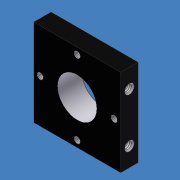
# Autodesk Inventor part: BB2-FrontPlate
Saved by Autodesk Inventor 2012 (Build 160160000, 160)
## iProperties
Company: FirstCadLibrary
Shininess: 64.0
Length Units: 11269
Angle Units: 11279
Time Units: 11290
Mass Units: 11283
Length Display Precision: 3
Angle Display Precision: 2
Compacted: True
Part Number: BB2-FrontPlate
Document SubType Name: Modeling
Created: 2007-01-08
Designer: Ed Sparks
Material: Aluminum-6061-AHC
Catalog Web Link: www.banebots.com
Vendor: BaneBots
Mass: 132.736 g
Surface Area: 141.952 cm^2
Volume: 48.98 cm^3
Density: 2.71 g/cm^3
Density: 0.0
Volumn: 0.0
Area: 0.0
PropertySet Name: Model Information
Control State: 0
Master: False
Checked Out: False
Author: Ed Sparks
Autodesk Inventor part; units mm, degrees
ref_plane "YZ Plane" through (0, 0, 0) normal (1, 0, 0) x (0, 1, 0)
ref_plane "XZ Plane" through (0, 0, 0) normal (0, 1, 0) x (-1, 0, 0)
sketch "Sketch1" plane through (0, 0, 0) normal (0, 0, 1) x (1, 0, 0)
  line L0 (-31.75, 31.75) -> (31.75, 31.75)
  line L1 (31.75, 31.75) -> (31.75, -31.75)
  line L2 (31.75, -31.75) -> (-31.75, -31.75)
  line L3 (-31.75, -31.75) -> (-31.75, 31.75)
  line L4 (0, 0) -> (0, 31.75) construction
  line L5 (0, 0) -> (0, -31.75) construction
  line L6 (0, 0) -> (31.75, 0) construction
  line L7 (0, 0) -> (-31.75, 0) construction
  dimension "d0" = 63.5
  dimension "d1" = 63.5
  constraints: 16 end point, 4 midpoint, 2 collinear, 2 parallel, 1 horizontal, 1 perpendicular, 1 other
  measures "d0" distance of L0.end L1.end
  measures "d1" distance of L0.start L0.end
extrude "Extrusion1" add sketch "Sketch1" along normal mid plane 12.7
sketch "Sketch6" plane through (0, 0, -6.35) normal (0, 0, -1) x (-1, 0, 0)
  circle A0 centre (0, 0) radius 25
  dimension "d13" = 50
  constraints: 1 centre point
  measures "d13" diameter of A0
extrude "Extrusion4" add sketch "Sketch6" along normal blind 6
sketch "Sketch8" plane through (0, 0, -12.35) normal (0, 0, -1) x (-1, 0, 0)
  circle A0 centre (0, 0) radius 25 projected
  constraints: 1 coincident
hole "Hole2" at (0, 0, -12.35) direction (0, 0, 1) diameter 28.575 end through all
chamfer "Chamfer1" distance 1 angle 45 1 edges at (0, -14.2875, -12.35)
sketch "Sketch9" plane through (-31.75, -31.75, 6.35) normal (0, -1, 0) x (1, 0, 0)
  line L0 (63.5, 0) -> (0, 0) projected
  line L1 (0, 0) -> (0, -12.7) projected
  line L2 (0, -12.7) -> (63.5, -12.7) projected
  line L3 (63.5, 0) -> (63.5, -12.7) projected
  line L4 (0, -6.35) -> (63.5, -6.35) construction
  line L5 (31.75, 0) -> (31.75, -12.7) construction
  point P0 (13.75, -6.35)
  dimension "d37" = 18
  constraints: 4 end point, 4 midpoint, 1 point on line
  measures "d37" distance from line of point (13.75, -6.35) L5
hole "Hole3" at (-18, -31.75, 0) direction (0, 1, 0) diameter 4.978 depth 13.7 tip angle 118 thread size "1/4-20 UNC" class "1B" standard "ANSI Unified Screw Threads"
mirror "Mirror1" about plane through (0, 0, 0) normal (1, 0, 0) of "Hole3"
mirror "Mirror2" about plane through (0, 0, 0) normal (0, 1, 0) of "Hole3", "Mirror1"
chamfer "Chamfer2" distance 1 angle 45 4 edges at (-18, -31.75, 2.489) (18, -31.75, 2.489) (-18, 31.75, 2.489) (18, 31.75, 2.489)
ref_plane "Work Plane1" through (0, 25, 0) normal (0, 1, 0) x (-1, 0, 0)
sketch "Sketch10" plane through (0, 25, 0) normal (0, 1, 0) x (-1, 0, 0)
  line L0 (-31.75, -6.35) -> (31.75, -6.35) projected
  line L1 (0, -6.35) -> (0, -22.9157) construction
  point P0 (0, -9.85)
  dimension "d48" = 3.5
  constraints: 2 end point, 1 midpoint, 1 perpendicular, 1 point on line
  measures "d48" distance from line of point (0, -9.85) L0
hole "Hole4" at (0, 25, -9.85) direction (0, -1, 0) diameter 2.459 depth 7.5 tip angle 118 thread size "M3x0.5" class "6H" standard "ANSI Metric M Profile"
pattern_circular "Circular Pattern2" count 4 over 360 about axis through (0, 0, 79.3789) along (0, 0, -1) of "Hole4"
sketch "Sketch11" plane through (0, 0, 6.35) normal (0, 0, 1) x (1, 0, 0)
  circle A0 centre (0, 0) radius 14.2875 projected
  line L0 (31.75, -31.75) -> (-31.75, -31.75) projected
  line L1 (0, 0) -> (36.6411, 0) construction
  point P0 (26.9875, 0)
  dimension "d59" = 26.9875
  constraints: 2 end point, 1 parallel, 1 point on line
  measures "d59" distance of point (26.988, 0) L1.start
hole "Hole5" at (26.9875, 0, 6.35) direction (0, 0, -1) diameter 4.134 end through all thread size "M5x0.8" class "6H" standard "ANSI Metric M Profile"
pattern_circular "Circular Pattern3" count 4 over 360 about axis through (0, 0, 79.3789) along (0, 0, -1) of "Hole5"
chamfer "Chamfer3" distance 0.25 angle 45 4 edges at (26.9875, 2.067, 6.35) (-2.067, 26.9875, 6.35) (-26.9875, -2.067, 6.35) (2.067, -26.9875, 6.35)
body "Solid1"
